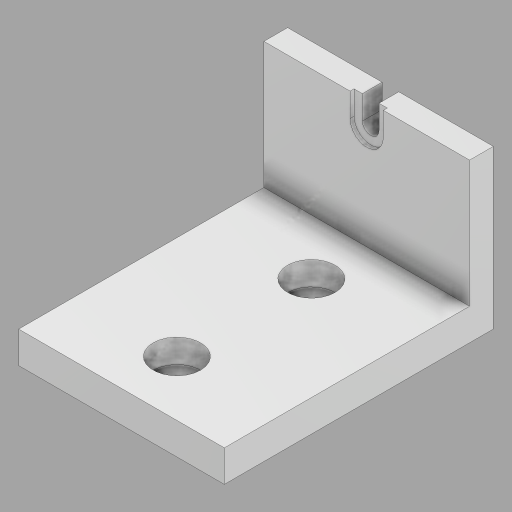
# Autodesk Inventor part: SupportSlide
Saved by Autodesk Inventor 2024 (Build 280153020, 153B)
## iProperties
Created: 2023-09-27
Part Number: SupportSlide
Material: Aluminum
Document SubType Name: Modeling
Designer: schanen
Density: 2.7 g/cm^3
Appearance: Satin
Author: schanen
Autodesk Inventor part; units mm, degrees
ref_plane "YZ Plane" through (0, 0, 0) normal (1, 0, 0) x (0, 1, 0)
ref_plane "XZ Plane" through (0, 0, 0) normal (0, 1, 0) x (-1, 0, 0)
ref_plane "XY Plane" through (0, 0, 0) normal (0, 0, 1) x (1, 0, 0)
sketch "Sketch1" plane through (0, 0, 0) normal (1, 0, 0) x (0, 1, 0)
  line L0 (20, 0) -> (20, 3)
  line L1 (20, 3) -> (4, 3)
  line L2 (4, 3) -> (4, 34)
  line L3 (4, 34) -> (0, 34)
  line L4 (0, 34) -> (0, 0)
  line L5 (0, 0) -> (20, 0)
  dimension "d0" = 3
  dimension "d1" = 4
  dimension "d2" = 34
  dimension "d3" = 20
  constraints: 12 end point, 5 perpendicular, 1 vertical
  measures "d0" distance of L0.start L0.end
  measures "d1" distance of L2.end L3.end
  measures "d2" distance of L3.end L4.end
  measures "d3" distance of L4.end L0.start
extrude "Extrusion1" add sketch "Sketch1" along normal blind 26
sketch "Sketch2" plane through (0, 4, 34) normal (0, 1, 0) x (1, 0, 0)
  line L0 (0, 31) -> (0, 0) projected
  line L1 (0, 0) -> (26, 0) projected
  line L2 (0, 31) -> (26, 31) projected
  point P0 (0, 34)
  point P1 (13, 7)
  point P2 (13, 24)
  dimension "d6" = 7
  dimension "d8" = 13
  dimension "d16" = 26
  dimension "d17" = 31
  dimension "d19" = 7
  constraints: 1 vertical alignment
  measures "d6" distance from line of L1 point (13, 7)
  measures "d8" distance from line of L0 point (13, 7)
  measures "d16" distance of L0.end L1.end
  measures "d17" distance of L0.start L0.end
  measures "d19" distance from line of L2 point (13, 24)
hole "Hole1" at (13, 4, 27) at (13, 4, 10) direction (0, -1, 0) diameter 2.459 end through all counterbore diameter 6 counterbore depth 3 thread size "M3x0.5" class "6H" standard "ISO Metric profile"
sketch "Sketch3" plane through (0, 4, 3) normal (0, 0, 1) x (1, 0, 0)
  line L0 (0, 16) -> (0, 0) projected
  line L1 (0, 16) -> (26, 16) projected
  circle A0 centre (13, 13) radius 1.05
  line L2 (11.95, 13) -> (11.95, 16)
  line L3 (14.05, 13) -> (14.05, 16)
  point P0 (0, -4)
  dimension "d20" = 2.1
  dimension "d21" = 13
  dimension "d22" = 3
  dimension "d28" = 26
  constraints: 4 end point, 2 perpendicular, 2 point on circle, 2 point on line, 2 tangent, 1 centre point
  measures "d20" diameter of A0
  measures "d21" distance from line of L0 A0.centre
  measures "d22" distance from line of L1 A0.centre
  measures "d28" distance of L0.start L1.end
extrude "Extrusion2" cut sketch "Sketch3" against normal through all
sketch "Sketch4" plane through (0, 4, 3) normal (0, 0, 1) x (1, 0, 0)
  arc A0 (11.95, 13) -> (14.05, 13) centre (13, 13) ccw projected
  circle A1 centre (13, 13) radius 2.1
  line L0 (0, 16) -> (11.95, 16) projected
  line L1 (14.05, 16) -> (26, 16) projected
  line L2 (10.9, 13) -> (10.9, 16)
  line L3 (15.1, 13) -> (15.1, 16)
  line L4 (10.9, 16) -> (15.1, 16)
  point P0 (0, -4)
  dimension "d25" = 4.2
  constraints: 6 end point, 2 perpendicular, 2 point on circle, 2 point on line, 2 tangent, 1 centre point, 1 coincident, 1 horizontal
  measures "d25" diameter of A1
extrude "Extrusion3" cut sketch "Sketch4" against normal blind 0.5
equation "\"d8\" = 0.5 * d16"
equation "\"d19\" = d6"
equation "\"d21\" = 0.5 * d28"
body "Solid1"
